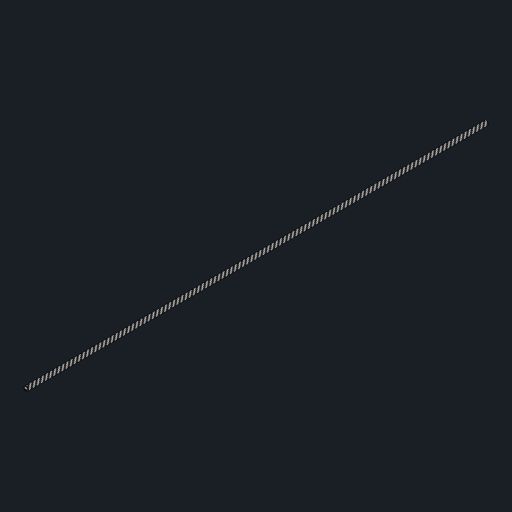
# Autodesk Inventor part: MainRod
Saved by Autodesk Inventor 2023 (Build 270158000, 158)
## iProperties
Created: 2022-07-08
Part Number: MainRod
Material: CFRP
Document SubType Name: Modeling
Designer: legot
Density: 1.43 g/cm^3
Appearance: カーボンファイバー
Author: legot
Autodesk Inventor part; units mm, degrees
ref_plane "YZ Plane" through (0, 0, 0) normal (1, 0, 0) x (0, 1, 0)
ref_plane "XZ Plane" through (0, 0, 0) normal (0, 1, 0) x (-1, 0, 0)
ref_plane "XY Plane" through (0, 0, 0) normal (0, 0, 1) x (1, 0, 0)
sketch "スケッチ1" plane through (0, 0, 0) normal (0, 0, 1) x (1, 0, 0)
  circle A0 centre (0, 0) radius 1.5
  line L0 (-2.8284, 0) -> (0, 2.8284)
  line L1 (0, 2.8284) -> (2.8284, 0)
  line L2 (2.8284, 0) -> (0, -2.8284)
  line L3 (0, -2.8284) -> (-2.8284, 0)
  dimension "d0" = 3
  dimension "d1" = 4
  constraints: 8 end point, 2 horizontal alignment, 2 parallel, 2 perpendicular, 1 centre point, 1 coincident, 1 vertical alignment
  measures "d0" diameter of A0
  measures "d1" distance of L0.start L0.end
extrude "押し出し1" add sketch "スケッチ1" against normal blind 420
